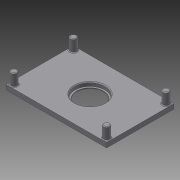
# Autodesk Inventor part: 37mm_sd_stage_insert
Saved by Autodesk Inventor 2013 (Build 170138000, 138)
## iProperties
Created: 2013-10-14
Part Number: 37mm_sd_stage_insert
Material: Generic
Document SubType Name: Modeling
Designer: kthorn
Density: 1 g/cm^3
Author: kthorn
Autodesk Inventor part; units mm, degrees
ref_plane "YZ Plane" through (0, 0, 0) normal (1, 0, 0) x (0, 1, 0)
ref_plane "XZ Plane" through (0, 0, 0) normal (0, 1, 0) x (-1, 0, 0)
ref_plane "XY Plane" through (0, 0, 0) normal (0, 0, 1) x (1, 0, 0)
sketch "Sketch1" plane through (0, 0, 0) normal (0, 0, 1) x (1, 0, 0)
  line L0 (63.85, 42.75) -> (-63.85, 42.75)
  line L1 (-63.85, 42.75) -> (-63.85, -42.75)
  line L2 (-63.85, -42.75) -> (63.85, -42.75)
  line L3 (63.85, -42.75) -> (63.85, 42.75)
  line L4 (63.85, 42.75) -> (-63.85, -42.75) construction
  line L5 (-63.85, 42.75) -> (63.85, -42.75) construction
  point P0 (0, 0)
  dimension "d0" = 85.5
  dimension "d2" = 127.7
  constraints: 12 end point, 2 midpoint, 2 parallel, 1 horizontal, 1 perpendicular
  measures "d0" distance of L0.end L1.end
  measures "d2" distance of L0.start L0.end
extrude "Extrusion1" add sketch "Sketch1" along normal blind 6
sketch "Sketch2" plane through (0, 0, 6) normal (0, 0, 1) x (1, 0, 0)
  circle A0 centre (0, 0) radius 19
  dimension "d5" = 38
  constraints: 1 centre point, 1 coincident
  measures "d5" diameter of A0
extrude "Extrusion2" cut sketch "Sketch2" against normal blind 5
sketch "Sketch3" plane through (0, 0, 1) normal (0, 0, 1) x (1, 0, 0)
  circle A0 centre (0, 0) radius 19 projected
  circle A1 centre (0, 0) radius 17
  dimension "d9" = 34
  constraints: 1 centre point, 1 coincident
  measures "d9" diameter of A1
extrude "Extrusion3" cut sketch "Sketch3" against normal through all contours A1
chamfer "Chamfer1" distance 1 angle 45 1 edges at (-19, 0, 6)
sketch "Sketch4" plane through (0, 0, 6) normal (0, 0, 1) x (1, 0, 0)
  line L0 (63.85, 42.75) -> (-63.85, 42.75) projected
  line L1 (-63.85, 42.75) -> (-63.85, -42.75) projected
  line L2 (-63.85, -42.75) -> (63.85, -42.75) projected
  line L3 (63.85, -42.75) -> (63.85, 42.75) projected
  line L4 (-63.85, 42.75) -> (-58.85, 42.75) construction
  line L5 (-58.85, 42.75) -> (-58.85, 37.75) construction
  circle A0 centre (-58.85, 37.75) radius 4
  line L6 (0, 42.75) -> (0, -42.75) construction
  line L7 (-63.85, 0) -> (63.85, 0) construction
  circle A1 centre (58.85, 37.75) radius 4
  circle A2 centre (-58.85, -37.75) radius 4
  circle A3 centre (58.85, -37.75) radius 4
  dimension "d16" = 5
  dimension "d18" = 8
  constraints: 8 end point, 4 centre point, 4 midpoint, 3 symmetric about line, 2 perpendicular, 1 coincident, 1 point on line, 3 other
  measures "d16" distance of L4.end L5.end
  measures "d18" diameter of A0
extrude "Extrusion4" add sketch "Sketch4" along normal blind 15 contours A0 | A1 | A2 | A3
fillet "Fillet1" radius 1 8 edges at (-62.85, 37.75, 6) (-62.85, 37.75, 21) (-62.85, -37.75, 21) (-62.85, -37.75, 6) (54.85, -37.75, 21) (54.85, -37.75, 6) (54.85, 37.75, 6) (54.85, 37.75, 21)
body "Solid1"
